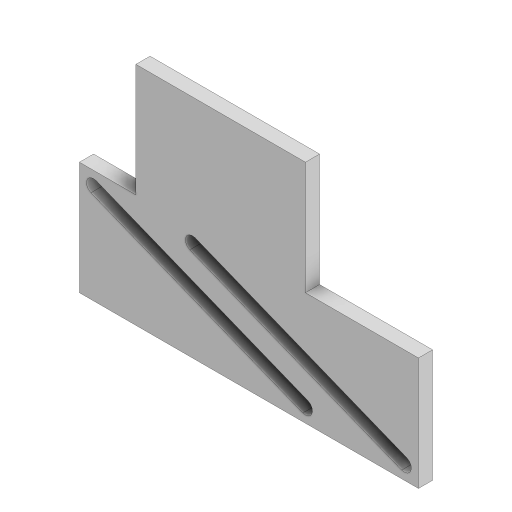
# Autodesk Inventor part: Short Wall Lift
Saved by Autodesk Inventor 2024.2 (Build 282272000, 272)
## iProperties
Created: 2024-12-02
Part Number: Short Wall Lift
Material: Generic
Document SubType Name: Modeling
Designer: rhond
Density: 1 g/cm^3
Appearance: Default
Author: rhond
Autodesk Inventor part; units mm, degrees
ref_plane "YZ Plane" through (0, 0, 0) normal (1, 0, 0) x (0, 1, 0)
ref_plane "XZ Plane" through (0, 0, 0) normal (0, 1, 0) x (-1, 0, 0)
ref_plane "XY Plane" through (0, 0, 0) normal (0, 0, 1) x (1, 0, 0)
sketch "Sketch2" plane through (0, 0, 0) normal (0, 0, 1) x (1, 0, 0)
  line L0 (0, 0) -> (76.2, 0)
  line L1 (76.2, 0) -> (76.2, 50.8)
  line L2 (76.2, 50.8) -> (0, 50.8)
  line L3 (0, 50.8) -> (0, 0)
  line L4 (-25.4, 0) -> (127, 0)
  line L5 (127, 0) -> (127, -50.8)
  line L6 (127, -50.8) -> (-25.4, -50.8)
  line L7 (-25.4, -50.8) -> (-25.4, 0)
  circle A0 centre (-19.05, -6.35) radius 3.175
  circle A1 centre (76.2, -44.45) radius 3.175
  line L8 (-17.8708, -3.4021) -> (77.3792, -41.5021)
  line L9 (-20.2292, -9.2979) -> (75.0208, -47.3979)
  circle A2 centre (25.4, -6.35) radius 3.175
  circle A3 centre (120.65, -44.45) radius 3.175
  line L10 (26.5792, -3.4021) -> (121.8292, -41.5021)
  line L11 (24.2208, -9.2979) -> (119.4708, -47.3979)
  dimension "d0" = 76.2
  dimension "d1" = 50.8
  dimension "d2" = 152.4
  dimension "d3" = 50.8
  dimension "d4" = 25.4
  dimension "d5" = 6.35
  dimension "d6" = 6.35
  dimension "d7" = 6.35
  dimension "d8" = 6.35
  dimension "d9" = 6.35
  dimension "d10" = 6.35
  dimension "d11" = 6.35
  dimension "d12" = 6.35
  constraints: 24 end point, 8 point on circle, 6 tangent, 4 centre point, 4 parallel, 3 horizontal, 2 perpendicular, 1 point on line
  measures "d0" distance of L2.end L1.end
  measures "d1" distance of L1.end L0.end
  measures "d2" distance of L5.end L6.end
  measures "d3" distance of L6.end L4.start
  measures "d4" distance between parallel lines of L7 L3
  measures "d5" diameter of A0
  measures "d6" distance from line of L4 A0.centre
  measures "d7" distance from line of L7 A0.centre
  measures "d8" diameter of A1
  measures "d9" distance from line of L6 A1.centre
  measures "d10" diameter of A2
  measures "d11" diameter of A3
  measures "d12" distance from line of L5 A3.centre
extrude "Extrusion1" add sketch "Sketch2" along normal blind 6.35
body "Solid1"
